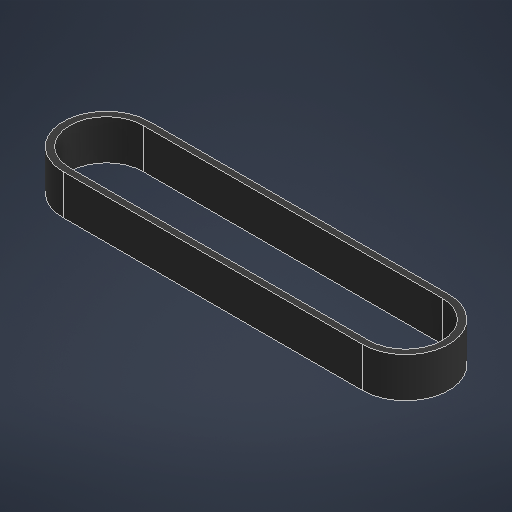
# Autodesk Inventor part: Timing belt
Saved by Autodesk Inventor 2026.1 (Build 301233000, 233)
## iProperties
Created: 2025-02-26
Part Number: Timing belt
Material: Generisch
Document SubType Name: Modeling
Designer: Luka Steib
Density: 1 g/cm^3
Appearance: Gummi - Schwarz
Author: Luka Steib
Autodesk Inventor part; units mm, degrees
ref_plane "YZ Plane" through (0, 0, 0) normal (1, 0, 0) x (0, 1, 0)
ref_plane "XZ Plane" through (0, 0, 0) normal (0, 1, 0) x (-1, 0, 0)
ref_plane "XY Plane" through (0, 0, 0) normal (0, 0, 1) x (1, 0, 0)
sketch "Skizze1" plane through (0, 0, 0) normal (0, 0, 1) x (1, 0, 0)
  line L0 (0, 0) -> (-44.947, 0) construction
  line L1 (0, 5.5) -> (-44.947, 5.5)
  line L2 (-44.947, -5.5) -> (0, -5.5)
  arc A0 (0, -5.5) -> (0, 5.5) centre (0, 0) ccw
  arc A1 (-44.947, 5.5) -> (-44.947, -5.5) centre (-44.947, 0) ccw
  line L3 (0, 0) -> (-44.947, 0) construction
  line L4 (0, -6.5) -> (-44.947, -6.5)
  line L5 (-44.947, 6.5) -> (0, 6.5)
  arc A2 (0, -6.5) -> (0, 6.5) centre (0, 0) ccw
  arc A3 (-44.947, 6.5) -> (-44.947, -6.5) centre (-44.947, 0) ccw
  point P0 (-22.4735, 0)
  point P1 (-22.4735, 0)
  dimension "d2" = 13
  dimension "d3" = 11
  dimension "d4" = 44.947
  constraints: 16 end point, 8 point on circle, 8 tangent, 4 centre point, 3 equal length, 2 midpoint, 1 horizontal
  measures "d2" distance between parallel lines of L4 L5
  measures "d3" distance between parallel lines of L2 L1
  measures "d4" distance of L0.start L0.end
extrude "Extrusion1" add sketch "Skizze1" along normal blind 6
